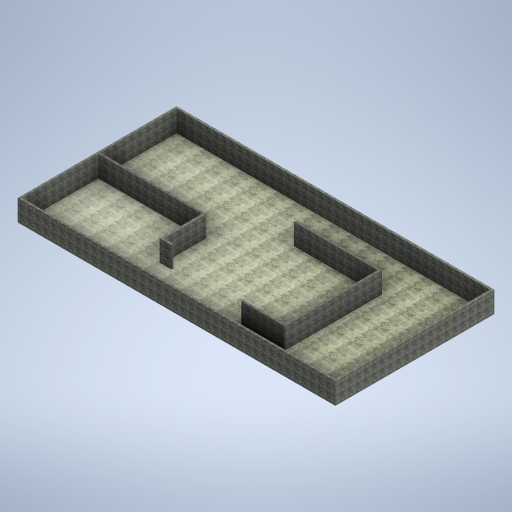
# Autodesk Inventor part: room
Saved by Autodesk Inventor 2024 (Build 280153000, 153)
## iProperties
Created: 2024-04-17
Part Number: room
Material: Generico
Document SubType Name: Modeling
Designer: matte
Density: 1 g/cm^3
Appearance: Default
Author: matte
Autodesk Inventor part; units mm, degrees
ref_plane "YZ Plane" through (0, 0, 0) normal (1, 0, 0) x (0, 1, 0)
ref_plane "XZ Plane" through (0, 0, 0) normal (0, 1, 0) x (-1, 0, 0)
ref_plane "XY Plane" through (0, 0, 0) normal (0, 0, 1) x (1, 0, 0)
sketch "Schizzo1" plane through (0, 0, 0) normal (0, 1, 0) x (-1, 0, 0)
  line L0 (-15000, 7500) -> (15000, 7500)
  line L1 (15000, 7500) -> (15000, -7500)
  line L2 (15000, -7500) -> (-15000, -7500)
  line L3 (-15000, -7500) -> (-15000, 7500)
  line L4 (-15000, 7500) -> (15000, -7500) construction
  line L5 (15000, 7500) -> (-15000, -7500) construction
  point P0 (0, 0)
  dimension "d0" = 30000
  dimension "d1" = 15000
  constraints: 12 end point, 2 midpoint, 2 parallel, 1 horizontal, 1 perpendicular
  measures "d0" distance of L1.end L2.end
  measures "d1" distance of L0.end L1.end
extrude "Estrusione1" add sketch "Schizzo1" against normal blind 10
sketch "Schizzo2" plane through (0, 0, 0) normal (0, 1, 0) x (1, 0, 0)
  line L0 (15000, 7500) -> (-15000, 7500) projected
  line L1 (-15000, 7500) -> (-15000, -7500) projected
  line L2 (-15000, -7500) -> (15000, -7500) projected
  line L3 (15000, -7500) -> (15000, 7500) projected
  line L4 (-5000, -100) -> (-5000, -4100)
  line L5 (-5000, -4100) -> (-3900, -4100)
  line L6 (-4800, 100) -> (-4800, -3900)
  line L7 (-4800, -3900) -> (-3900, -3900)
  line L8 (-3900, -3900) -> (-3900, -4100)
  line L9 (0, 3800) -> (8100, 3800)
  line L10 (8100, 3800) -> (8100, -5400)
  line L11 (8100, -5400) -> (4000, -5400)
  line L12 (4000, -5200) -> (7900, -5200)
  line L13 (7900, -5200) -> (7900, 3600)
  line L14 (7900, 3600) -> (0, 3600)
  line L15 (0, 3800) -> (0, 3600)
  line L16 (4000, -5200) -> (4000, -5400)
  line L17 (-14800, 7300) -> (14800, 7300)
  line L18 (14800, 7300) -> (14800, -7300)
  line L19 (14800, -7300) -> (-14800, -7300)
  line L20 (-14800, -7300) -> (-14800, 7300)
  line L21 (-4800, 100) -> (-14800, 100)
  line L22 (-5000, -100) -> (-14800, -100)
  line L23 (-15000, 7500) -> (15000, 7500)
  line L24 (15000, 7500) -> (15000, -7500)
  line L25 (15000, -7500) -> (-15000, -7500)
  line L26 (-15000, -7500) -> (-15000, 7500)
  point P0 (0, 0)
  constraints: 46 end point, 4 parallel, 2 perpendicular, 2 point on line, 2 vertical, 1 horizontal, 3 other
extrude "Estrusione2" add sketch "Schizzo2" along normal blind 2000 contours L3 L2 L1 L0 | L22 L20 L21 L6 L7 L8 L5 L4 | L9 L10 L11 L16 L12 L13 L14 L15
